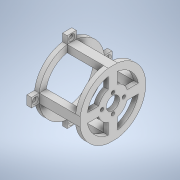
# Autodesk Inventor part: Gear_Box_Motor_Support_Bracket
Saved by Autodesk Inventor 2022 (Build 260153000, 153)
## iProperties
Created: 2022-04-22
Part Number: Gear_Box_Motor_Support_Bracket
Material: Generic
Document SubType Name: Modeling
Designer: Mlees
Density: 1 g/cm^3
Appearance: Default
Author: Mlees
Autodesk Inventor part; units mm, degrees
ref_plane "YZ Plane" through (0, 0, 0) normal (1, 0, 0) x (0, 1, 0)
ref_plane "XZ Plane" through (0, 0, 0) normal (0, 1, 0) x (-1, 0, 0)
ref_plane "XY Plane" through (0, 0, 0) normal (0, 0, 1) x (1, 0, 0)
sketch "Sketch1" plane through (0, 0, 0) normal (1, 0, 0) x (0, 1, 0)
  line L0 (28.3441, -4) -> (35, -4)
  line L1 (28.3441, 4) -> (35, 4)
  line L2 (35, 4) -> (35, -4)
  circle A0 centre (31.6721, 0) radius 1.625
  line L3 (-4, 28.3441) -> (-4, 35)
  circle A1 centre (0, 31.6721) radius 1.625
  line L4 (-4, 35) -> (4, 35)
  line L5 (4, 28.3441) -> (4, 35)
  line L6 (-28.3441, -4) -> (-35, -4)
  circle A2 centre (-31.6721, 0) radius 1.625
  line L7 (-35, -4) -> (-35, 4)
  line L8 (-28.3441, 4) -> (-35, 4)
  line L9 (4, -28.3441) -> (4, -35)
  circle A3 centre (0, -31.6721) radius 1.625
  line L10 (4, -35) -> (-4, -35)
  line L11 (-4, -28.3441) -> (-4, -35)
  arc A4 (28.3441, 4) -> (4, 28.3441) centre (0, 0) ccw
  arc A5 (-4, 28.3441) -> (-28.3441, 4) centre (0, 0) ccw
  arc A6 (-28.3441, -4) -> (-4, -28.3441) centre (0, 0) ccw
  arc A7 (4, -28.3441) -> (28.3441, -4) centre (0, 0) ccw
  circle A8 centre (0, 0) radius 22.5
  dimension "d4" = 3.25
  dimension "d7" = 360
  constraints: 24 end point, 9 centre point, 8 point on circle, 2 coincident, 1 perpendicular, 37 other
  measures "d4" diameter of A0
extrude "Extrusion1" add sketch "Sketch1" along normal blind 4
sketch "Sketch2" plane through (4, 0, 0) normal (1, 0, 0) x (0, 0, -1)
  line L0 (4, 28.3441) -> (4, 35) projected
  line L1 (-4, 28.3441) -> (4, 28.3441)
  line L2 (4, 28.3441) -> (4, 22.1416)
  circle A0 centre (0, 0) radius 22.5 projected
  line L3 (-4, 22.1416) -> (-4, 28.3441)
  arc A1 (-4, 28.3441) -> (-28.3441, 4) centre (0, 0) ccw projected
  line L4 (-28.3441, -4) -> (-28.3441, 4)
  line L5 (-28.3441, 4) -> (-22.1416, 4)
  line L6 (-35, -4) -> (-28.3441, -4) projected
  line L7 (-28.3441, -4) -> (-22.1416, -4)
  line L8 (4, -35) -> (4, -28.3441) projected
  line L9 (-4, -28.3441) -> (4, -28.3441)
  line L10 (4, -28.3441) -> (4, -22.1416)
  line L11 (-4, -28.3441) -> (-4, -22.1416)
  arc A2 (28.3441, 4) -> (4, 28.3441) centre (0, 0) ccw projected
  line L12 (28.3441, -4) -> (28.3441, 4)
  line L13 (28.3441, 4) -> (22.1416, 4)
  line L14 (28.3441, -4) -> (22.1416, -4)
  arc A3 (4, 22.1416) -> (-4, 22.1416) centre (0, 0) ccw
  arc A4 (22.1416, -4) -> (22.1416, 4) centre (0, 0) ccw
  arc A5 (-4, -22.1416) -> (4, -22.1416) centre (0, 0) ccw
  arc A6 (-22.1416, 4) -> (-22.1416, -4) centre (0, 0) ccw
  constraints: 24 end point, 8 point on circle, 4 centre point, 3 perpendicular, 2 horizontal, 2 parallel, 2 point on line, 2 vertical, 1 collinear, 13 other
extrude "Extrusion2" add sketch "Sketch2" along normal blind 31.725 contours L1 L2 A0 L3 | L5 A0 L7 L4 | L12 L14 A0 L13 | A0 L10 L9 L11
sketch "Sketch3" plane through (35.725, 0, 0) normal (1, 0, 0) x (0, 0, -1)
  line L0 (-4, 28.3441) -> (4, 28.3441) projected
  line L1 (28.3441, -4) -> (28.3441, 4) projected
  line L2 (28.3441, 4) -> (28.3441, -4)
  arc A0 (28.3441, 4) -> (4, 28.3441) centre (0, 0) ccw
  line L3 (-4, -28.3441) -> (4, -28.3441) projected
  line L4 (4, -28.3441) -> (-4, -28.3441)
  arc A1 (4, -28.3441) -> (28.3441, -4) centre (0, 0) ccw
  line L5 (-35, -4) -> (-28.3441, -4) projected
  line L6 (-28.3441, 4) -> (-28.3441, -4) projected
  line L7 (-28.3441, -4) -> (-28.3441, 4)
  arc A2 (-4, 28.3441) -> (-28.3441, 4) centre (0, 0) ccw
  arc A3 (-28.3441, -4) -> (-4, -28.3441) centre (0, 0) ccw
  circle A4 centre (0, 0) radius 5.715
  circle A5 centre (9.4996, 0) radius 1.4986
  circle A6 centre (-9.4996, 0) radius 1.4986
  circle A7 centre (0, 8.001) radius 1.4986
  circle A8 centre (0, -8.001) radius 1.4986
  line L8 (-4, 22.1416) -> (-4, 28.3441) projected
  line L9 (4, 28.3441) -> (4, 22.1416) projected
  line L10 (4, 12.3744) -> (4, 22.1416)
  line L11 (-4, 22.1416) -> (-4, 12.3744)
  line L12 (-4, 28.3441) -> (4, 28.3441)
  line L13 (28.3441, 4) -> (22.1416, 4) projected
  line L14 (22.1416, 4) -> (12.3744, 4)
  arc A9 (4, -28.3441) -> (28.3441, -4) centre (0, 0) ccw projected
  line L15 (22.1416, -4) -> (12.3744, -4)
  line L16 (4, -22.1416) -> (4, -12.3744)
  arc A10 (-28.3441, -4) -> (-4, -28.3441) centre (0, 0) ccw projected
  line L17 (-4, -22.1416) -> (-4, -12.3744)
  line L18 (-22.1416, -4) -> (-12.3744, -4)
  arc A11 (-4, 28.3441) -> (-28.3441, 4) centre (0, 0) ccw projected
  line L19 (-22.1416, 4) -> (-12.3744, 4)
  arc A12 (-4, 12.3744) -> (-12.3744, 4) centre (0, 0) ccw
  arc A13 (-4, 22.1416) -> (-22.1416, 4) centre (0, 0) ccw
  arc A14 (12.3744, 4) -> (4, 12.3744) centre (0, 0) ccw
  arc A15 (22.1416, 4) -> (4, 22.1416) centre (0, 0) ccw
  arc A16 (-22.1416, -4) -> (-4, -22.1416) centre (0, 0) ccw
  arc A17 (4, -22.1416) -> (22.1416, -4) centre (0, 0) ccw
  arc A18 (-12.3744, -4) -> (-4, -12.3744) centre (0, 0) ccw
  arc A19 (4, -12.3744) -> (12.3744, -4) centre (0, 0) ccw
  dimension "d17" = 11.43
  dimension "d18" = 2.9972
  dimension "d19" = 2.9972
  constraints: 26 end point, 24 point on circle, 17 centre point, 6 collinear, 3 coincident, 3 point on line, 1 parallel, 1 perpendicular, 1 vertical
  measures "d17" diameter of A4
  measures "d18" diameter of A5
  measures "d19" diameter of A7
extrude "Extrusion3" add sketch "Sketch3" along normal blind 4 contours L0 L9 L10 A14 L14 L13 L1 A1 L3 A3 L6 A2 | A0 L13 A15 L9
chamfer "Chamfer1" distance 1.1 angle 45 4 edges at (4, 30.0471, 0) (4, -1.625, -31.6721) (4, -33.2971, 0) (4, -1.625, 31.6721)
body "Solid1"
